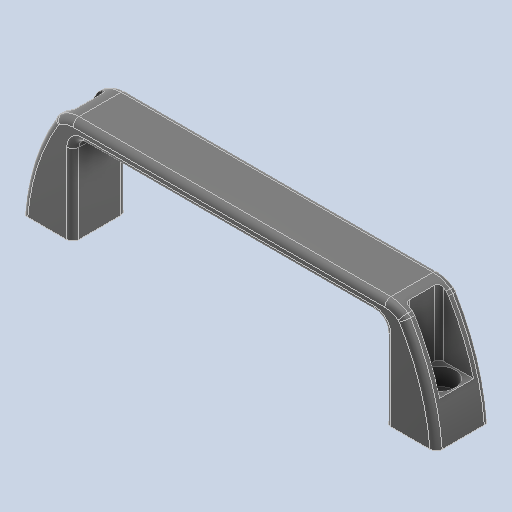
# Autodesk Inventor part: Handle
Saved by Autodesk Inventor 2026.2 (Build 302298000, 298)
## iProperties
Created: 2025-07-30
Part Number: Handle
Material: Acetal Resin, Black
Document SubType Name: Modeling
Designer: mumin
Density: 1.425 g/cm^3
Appearance: Smooth - Black
Author: mumin
Autodesk Inventor part; units mm, degrees
ref_plane "YZ Plane" through (0, 0, 0) normal (1, 0, 0) x (0, 1, 0)
ref_plane "XZ Plane" through (0, 0, 0) normal (0, 1, 0) x (-1, 0, 0)
ref_plane "XY Plane" through (0, 0, 0) normal (0, 0, 1) x (1, 0, 0)
sketch "Sketch1" plane through (0, 0, 0) normal (0, 0, 1) x (1, 0, 0)
  line L0 (0.057, 44) -> (71, 44)
  line L1 (76.057, 52) -> (0.057, 52)
  line L2 (101.057, 0) -> (76, 0)
  line L3 (76, 0) -> (76, 39)
  arc A0 (101.057, 0) -> (85.6787, 47.8152) centre (-6.9827, -8.3672) ccw
  arc A1 (84.3966, 49.2278) -> (76.057, 52) centre (76.057, 38.0701) ccw
  arc A2 (85.6787, 47.8152) -> (84.3966, 49.2278) centre (81.4032, 45.2229) ccw
  line L4 (0.057, 44) -> (-71, 44)
  line L5 (-75.943, 52) -> (0.057, 52)
  line L6 (-100.943, 0) -> (-76, 0)
  line L7 (-76, 0) -> (-76, 39)
  arc A3 (-85.5646, 47.8152) -> (-100.943, 0) centre (7.0967, -8.3672) ccw
  arc A4 (-75.943, 52) -> (-84.2825, 49.2278) centre (-75.943, 38.0701) ccw
  arc A5 (-84.2825, 49.2278) -> (-85.5646, 47.8152) centre (-81.2891, 45.2229) ccw
  arc A6 (76, 39) -> (71, 44) centre (71, 39) ccw
  arc A7 (-71, 44) -> (-76, 39) centre (-71, 39) ccw
  line L8 (0, -20.5757) -> (0, 64.8833) projected
  point P0 (0, 0)
  point P1 (76, 44)
  point P2 (0.1141, 0)
  point P3 (-76, 44)
  dimension "d1" = 44
  dimension "d2" = 8
  dimension "d4" = 5
  dimension "d5" = 152
  dimension "d10" = 5
  constraints: 16 end point, 16 point on circle, 8 centre point, 7 tangent, 6 point on line, 1 equal radius, 1 horizontal, 1 parallel, 1 other
  measures "d1" distance from line of point (0, 0) L0
  measures "d2" distance between parallel lines of L1 L0
  measures "d4" radius of A2
  measures "d5" distance between parallel lines of L3 L7
  measures "d10" radius of A6
extrude "Extrusion1" add sketch "Sketch1" along normal mid plane 26.5
fillet "Fillet1" radius 3 14 edges at (-80.3371, 51.2888, 13.25) (-84.9915, 48.5832, 13.25) (-96.0624, 24.8109, 13.25) (80.4512, 51.2888, 13.25) (85.1056, 48.5832, 13.25) (96.1764, 24.8109, 13.25) (0.057, 52, 13.25) (80.4512, 51.2888, -13.25) (85.1056, 48.5832, -13.25) (96.1764, 24.8109, -13.25) (-80.3371, 51.2888, -13.25) (-84.9915, 48.5832, -13.25) (-96.0624, 24.8109, -13.25) (0.057, 52, -13.25)
fillet "Fillet2" radius 3 6 edges at (0, 44, 13.25) (76, 19.5, 13.25) (-76, 19.5, 13.25) (-76, 19.5, -13.25) (0, 44, -13.25) (76, 19.5, -13.25)
sketch "Sketch2" plane through (-75.943, 52, -10.25) normal (0, 1, 0) x (1, 0, 0)
  line L0 (-0.057, 0) -> (-0.057, -20.5) projected
  line L1 (151.943, 0) -> (151.943, -20.5) projected
  line L2 (177, 0) -> (177, -20.5) projected
  line L3 (177, -2) -> (158.943, -2)
  line L4 (156.943, -4) -> (156.943, -16.5)
  line L5 (158.943, -18.5) -> (177, -18.5)
  line L6 (177, -18.5) -> (177, -2)
  line L7 (159.0563, 3) -> (173.9908, 3) projected
  line L8 (173.9908, -23.5) -> (159.0563, -23.5) projected
  arc A0 (158.943, -2) -> (156.943, -4) centre (158.943, -4) ccw
  arc A1 (156.943, -16.5) -> (158.943, -18.5) centre (158.943, -16.5) ccw
  line L9 (-25, 0) -> (-25, -20.5) projected
  line L10 (-25, -2) -> (-7.057, -2)
  line L11 (-5.057, -4) -> (-5.057, -16.5)
  line L12 (-7.057, -18.5) -> (-25, -18.5)
  line L13 (-25, -18.5) -> (-25, -2)
  arc A2 (-5.057, -4) -> (-7.057, -2) centre (-7.057, -4) ccw
  arc A3 (-7.057, -18.5) -> (-5.057, -16.5) centre (-7.057, -16.5) ccw
  point P0 (75.943, -10.25)
  point P1 (166.5236, 3)
  dimension "d11" = 5
  dimension "d12" = 5
  dimension "d13" = 5
  dimension "d14" = 2
  dimension "d15" = 5
  dimension "d16" = 2
  constraints: 16 end point, 8 point on circle, 8 tangent, 4 centre point, 4 parallel, 2 equal radius, 2 horizontal, 2 perpendicular, 2 point on line, 1 midpoint
  measures "d11" distance between parallel lines of L4 L1
  measures "d12" distance from line of L3 point (166.524, 3)
  measures "d13" distance between parallel lines of L8 L5
  measures "d14" radius of A0
  measures "d15" distance between parallel lines of L0 L11
  measures "d16" radius of A2
extrude "Extrusion2" cut sketch "Sketch2" against normal blind 33
sketch "Sketch3" plane through (-75.943, 19, -10.25) normal (0, 1, 0) x (1, 0, 0)
  line L0 (-65.4065, -10.25) -> (217.4065, -10.25) projected
  line L1 (-5.057, -4) -> (-5.057, -16.5) projected
  line L2 (75.943, 8.3065) -> (75.943, -28.8065) projected
  point P0 (75.943, -10.25)
  point P1 (-13.751, -10.25)
  dimension "d27" = 89.694
  constraints: 1 point on line
  measures "d27" distance from line of point (-13.751, -10.25) L2
hole "Hole1" at (-89.694, 19, 0) direction (0, -1, 0) diameter 8 end through all counterbore diameter 15 counterbore depth 8.6
mirror "Mirror1" about plane through (0, 0, 0) normal (1, 0, 0) of "Hole1"
body "Solid1"
